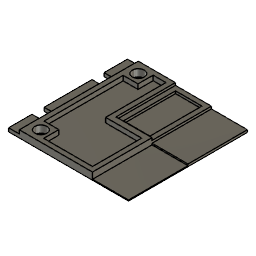
3D Filament Swatch-60103-PC-Transparent (Autodesk Fusion 360 design; units mm, degrees)
Autodesk Fusion 360 part; units mm, degrees
sketch "Schizzo1" plane through (0, 0, 0) normal (0, 0, 1) x (1, 0, 0)
  line L0 (39.1195, 62.1228) -> (89.1195, 62.1228)
  line L1 (89.1195, 62.1228) -> (89.1195, 12.5228)
  line L2 (89.1195, 12.5228) -> (39.1195, 12.5228)
  line L3 (39.1195, 12.5228) -> (39.1195, 62.1228)
  line L4 (43.6195, 62.1228) -> (43.6195, 12.5228)
  line L5 (74.1195, 62.1228) -> (74.1195, 12.5228)
  line L6 (39.1195, 37.3228) -> (89.1195, 37.3228) construction
  line L7 (48.1195, 62.1228) -> (48.1195, 12.5228) construction
  circle A0 centre (48.1195, 57.6228) radius 2.5
  circle A1 centre (48.1195, 17.0228) radius 2.5
  line L8 (74.1195, 37.3228) -> (89.1195, 37.3228)
  line L9 (86.071, 62.1228) -> (86.071, 12.5228) construction
  line L10 (59.1195, 62.1228) -> (59.1195, 37.3228)
  line L11 (74.1195, 37.3228) -> (59.1195, 37.3228)
  line L12 (39.1195, 52.3228) -> (43.6195, 52.3228)
  line L13 (43.6195, 52.3228) -> (43.6195, 47.3228)
  line L14 (43.6195, 47.3228) -> (39.1195, 47.3228)
  line L15 (39.1195, 47.3228) -> (39.1195, 52.3228)
  line L16 (43.6195, 27.3228) -> (39.1195, 27.3228)
  line L17 (39.1195, 22.3228) -> (43.6195, 22.3228)
  line L18 (39.1195, 49.8228) -> (43.6195, 49.8228) construction
  line L19 (39.1195, 24.8228) -> (43.6195, 24.8228) construction
  dimension "d1" = 50
  dimension "d2" = 49.6
  dimension "d3" = 4.5
  dimension "d4" = 15
  dimension "d6" = 5
  dimension "d7" = 40.6
  dimension "d26" = 9
  dimension "d29" = 15
  dimension "d40" = 5
  dimension "d41" = 25
  constraint horizontal L0
  constraint vertical L1
  constraint horizontal L2
  constraint vertical L3
  constraint coincident L0 L4.start
  constraint coincident L2 L4.end
  constraint perpendicular L2 L4
  constraint coincident L0 L5.start
  constraint coincident L2 L5.end
  constraint perpendicular L2 L5
  constraint midpoint L3 L6.start
  constraint midpoint L1 L6.end
  constraint coincident L0 L7.start
  constraint coincident L2 L7.end
  constraint perpendicular L2 L7
  constraint coincident L7 A0.centre
  constraint symmetric L6 A0 A1
  constraint midpoint L5 L8.start
  constraint coincident L0 L9.start
  constraint coincident L2 L9.end
  constraint perpendicular L2 L9
  constraint coincident L0 L10.start
  constraint coincident L6 L10.end
  constraint perpendicular L6 L10
  constraint perpendicular L10 L11
  constraint horizontal L12
  constraint vertical L13
  constraint horizontal L14
  constraint vertical L15
  constraint coincident L3 L12.start
  constraint symmetric L6 L12.start L17.start
  constraint symmetric L6 L12.end L17.end
  constraint symmetric L6 L13.end L16.start
  constraint symmetric L6 L14.end L16.end
  constraint midpoint L15 L18.start
  constraint midpoint L13 L18.end
  constraint symmetric L6 L18.start L19.start
  constraint symmetric L6 L18.end L19.end
  measures "d1" distance of L0.start L0.end
  measures "d2" distance of L0.start L2.end
  measures "d3" distance of L3 L4
  measures "d4" distance of L1 L5
  measures "d6" diameter of A0
  measures "d7" distance of A0.centre A1.centre
  measures "d26" distance of L3 L7
  measures "d29" distance of L5 L10
  measures "d40" distance of L12.start L14.end
  measures "d41" distance of L18 L19
extrude "Estrusione1" add sketch "Schizzo1" along normal blind 3 contours L0 L2 L4 L5 L10 L11 L13
extrude "Estrusione7" add sketch "Schizzo1" along normal blind 2 contours L0 L5 L10 L11
extrude "Estrusione2" add sketch "Schizzo1" along normal blind 0.4 contours L1 L2 L5 L8
extrude "Estrusione6" add sketch "Schizzo1" along normal blind 1 contours L0 L1 L5 L8
extrude "Estrusione3" add sketch "Schizzo1" along normal blind 1.5 contours L0 L3 L4 L12 | L3 L4 L14 L16 | L2 L3 L4 L17
sketch "Schizzo4" plane through (0, 0, 3) normal (0, 0, 1) x (-1, 0, 0)
  circle A0 centre (-48.1195, -57.6228) radius 2.5
  circle A1 centre (-48.1195, -17.0228) radius 2.5
  line L0 (-74.1195, -12.5228) -> (-74.1195, -37.3228)
  line L1 (-74.1195, -37.3228) -> (-59.1195, -37.3228)
  line L2 (-59.1195, -37.3228) -> (-59.1195, -62.1228)
  line L3 (-59.1195, -62.1228) -> (-43.6195, -62.1228)
  line L4 (-43.6195, -62.1228) -> (-43.6195, -12.5228)
  line L5 (-43.6195, -12.5228) -> (-74.1195, -12.5228)
  line L6 (-59.1195, -37.3228) -> (-45.6195, -37.3228) construction
  line L7 (-51.7809, -60.1228) -> (-57.1195, -60.1228)
  line L8 (-57.1195, -60.1228) -> (-57.1195, -35)
  line L9 (-57.1195, -35) -> (-72.1195, -35)
  line L10 (-72.1195, -35) -> (-72.1195, -14.5228)
  line L11 (-72.1195, -14.5228) -> (-51.7809, -14.5228)
  line L12 (-51.7809, -14.5228) -> (-51.7809, -20.8228)
  line L13 (-51.7809, -20.8228) -> (-45.6195, -20.8228)
  line L14 (-45.6195, -20.8228) -> (-45.6195, -53.8228)
  line L15 (-45.6195, -53.8228) -> (-51.7809, -53.8228)
  line L16 (-51.7809, -53.8228) -> (-51.7809, -60.1228)
  point P0 (-45.6195, -37.3228)
  dimension "d47" = 2
  dimension "d48" = 2
  dimension "d49" = 2
  dimension "d50" = 2
  dimension "d51" = 2
  dimension "d52" = 33
  constraint coincident L1.end L2.start
  constraint horizontal L7
  constraint perpendicular L6 L8
  constraint perpendicular L8 L9
  constraint perpendicular L9 L10
  constraint perpendicular L10 L11
  constraint perpendicular L11 L12
  constraint perpendicular L12 L13
  constraint perpendicular L13 L14
  constraint perpendicular L14 L15
  constraint perpendicular L15 L16
  constraint collinear L12 L16
  constraint coincident P0 L14
  constraint coincident P0 L6.end
  constraint equal L12 L16
  measures "d47" distance of L3 L7
  measures "d48" distance of L5 L11
  measures "d49" distance of L2 L8
  measures "d50" distance of L0 L10
  measures "d51" distance of L4 L14
  measures "d52" distance of L13 L15
sketch "Schizzo5" plane through (0, 0, 2) normal (0, 0, 1) x (-1, 0, 0)
  line L0 (-59.1195, -62.1228) -> (-59.1195, -37.3228)
  line L1 (-59.1195, -37.3228) -> (-74.1195, -37.3228)
  line L2 (-74.1195, -37.3228) -> (-74.1195, -62.1228)
  line L3 (-74.1195, -62.1228) -> (-59.1195, -62.1228)
  line L4 (-61.1195, -60.1228) -> (-72.1195, -60.1228)
  line L5 (-72.1195, -60.1228) -> (-72.1195, -38.4568)
  line L6 (-72.1195, -38.4568) -> (-61.1195, -38.4568)
  line L7 (-61.1195, -38.4568) -> (-61.1195, -60.1228)
  line L8 (-59.1195, -37.3228) -> (-59.1195, -62.1228)
  dimension "d42" = 2
  dimension "d43" = 2
  dimension "d44" = 2
  constraint horizontal L4
  constraint vertical L5
  constraint horizontal L6
  constraint vertical L7
  measures "d42" distance of L3 L4
  measures "d43" distance of L7 L8
  measures "d44" distance of L2 L5
sketch "Schizzo6" plane through (0, 0, 1) normal (0, 0, 1) x (-1, 0, 0)
  line L0 (-74.1195, -62.1228) -> (-74.1195, -37.3228)
  line L1 (-74.1195, -37.3228) -> (-89.1195, -37.3228)
  line L2 (-89.1195, -37.3228) -> (-89.1195, -62.1228)
  line L3 (-89.1195, -62.1228) -> (-74.1195, -62.1228)
extrude "Estrusione10" cut sketch "Schizzo5" against normal blind 1 contours L4 L5 L6 L7
extrude "Estrusione11" cut sketch "Schizzo4" against normal blind 2 contours L7 L8 L9 L10 L11 L12 L13 L14 L15 L16
extrude "Estrusione9" [suppressed]
extrude "Estrusione8" [suppressed]
equation "d2 = 50 mm - 0.4 mm"
equation "d7 = d2 - 9 mm"
named bodies: "Body"
